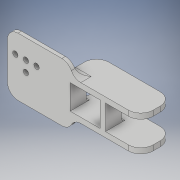
# Autodesk Inventor part: v5_tibia_B
Saved by Autodesk Inventor 2019 (Build 230136000, 136)
## iProperties
Created: 2019-01-20
Part Number: v5_tibia_B
Material: Generic
Document SubType Name: Modeling
Designer: Daniel
Density: 1 g/cm^3
Appearance: Default
Author: Daniel
Autodesk Inventor part; units mm, degrees
ref_plane "YZ Plane" through (0, 0, 0) normal (1, 0, 0) x (0, 1, 0)
ref_plane "XZ Plane" through (0, 0, 0) normal (0, 1, 0) x (-1, 0, 0)
ref_plane "XY Plane" through (0, 0, 0) normal (0, 0, 1) x (1, 0, 0)
sketch "Sketch1" plane through (0, 0, 0) normal (0, 1, 0) x (-1, 0, 0)
  line L0 (39, 2) -> (-3, 2)
  line L1 (-3, 2) -> (-3, 0)
  line L2 (-3, 0) -> (39, 0)
  line L3 (39, 0) -> (39, 2)
  line L4 (47.4, 0) -> (-11.4, 0) projected
  line L5 (0, -19.6) -> (0, 5.6) projected
  line L6 (0, -16) -> (-3, -16)
  line L7 (-3, -16) -> (-3, 0)
  line L8 (-3, 0) -> (0, 0)
  line L9 (0, 0) -> (0, -16)
  point P0 (0, 0)
  dimension "d0" = 2
  dimension "d1" = 3
  dimension "d2" = 42
  dimension "d3" = 18
  constraints: 16 end point, 4 collinear, 4 parallel, 2 horizontal, 2 perpendicular
  measures "d0" distance between parallel lines of L0 L2
  measures "d1" distance between parallel lines of L7 L9
  measures "d2" distance between parallel lines of L1 L3
  measures "d3" distance between parallel lines of L0 L6
extrude "Extrusion1" add sketch "Sketch1" along normal blind 33
sketch "Sketch2" plane through (-39, 0, 2) normal (0, 0, 1) x (1, 0, 0)
  line L0 (0, 0) -> (42, 0) projected
  line L1 (42, 0) -> (42, 33) projected
  line L2 (0, 33) -> (42, 33) projected
  line L3 (0, 0) -> (0, 33) projected
  point P0 (39, 0)
  point P1 (17, 11)
  point P2 (17, 17)
  point P3 (11, 11)
  point P4 (23, 11)
  dimension "d7" = 6
  dimension "d8" = 6
  dimension "d9" = 6
  dimension "d11" = 11
  dimension "d12" = 6
  dimension "d14" = 6
  dimension "d15" = 6
  dimension "d69" = 11
  measures "d7" distance of point (17, 11) point (17, 17)
  measures "d8" distance of point (17, 11) point (11, 11)
  measures "d9" distance of point (17, 11) point (23, 11)
  measures "d11" distance from line of L3 point (11, 11)
  measures "d12" horizontal distance of point (17, 17) point (11, 11)
  measures "d14" horizontal distance of point (17, 17) point (23, 11)
  measures "d15" horizontal distance of point (11, 11) point (17, 17)
  measures "d69" distance from line of L0 point (11, 11)
hole "Hole1" at (-22, 11, 2) at (-22, 17, 2) at (-28, 11, 2) at (-16, 11, 2) direction (0, 0, -1) diameter 3 end through all
sketch "Sketch9" plane through (3, 0, 2) normal (1, 0, 0) x (0, 0, -1)
  line L0 (18, 0) -> (0, 0) projected
  line L1 (18, 0) -> (18, 33) projected
  line L2 (0, 33) -> (18, 33) projected
  line L3 (0, 0) -> (0, 33) projected
  line L4 (2, 0) -> (2, 33) projected
  line L5 (0, 0) -> (0, 33) projected
  line L6 (0, 16.5) -> (18, 16.5) construction
  line L7 (0, 6.5) -> (18, 6.5)
  line L8 (18, 6.5) -> (18, 9.5)
  line L9 (18, 9.5) -> (0, 9.5)
  line L10 (0, 9.5) -> (0, 6.5)
  line L11 (0, 23.5) -> (18, 23.5)
  line L12 (18, 23.5) -> (18, 26.5)
  line L13 (18, 26.5) -> (0, 26.5)
  line L14 (0, 26.5) -> (0, 23.5)
  line L15 (0, 0) -> (0, 33) projected
  line L16 (18, 0) -> (18, 33) projected
  dimension "d81" = 16.5
  dimension "d82" = 3
  dimension "d83" = 3
  dimension "d84" = 7
  dimension "d85" = 7
  constraints: 18 end point, 4 parallel, 3 collinear, 3 perpendicular, 2 horizontal, 2 midpoint, 1 point on line
  measures "d81" distance between parallel lines of L2 L6
  measures "d82" distance between parallel lines of L13 L11
  measures "d83" distance between parallel lines of L7 L9
  measures "d84" distance between parallel lines of L6 L9
  measures "d85" distance between parallel lines of L11 L6
extrude "Extrusion6" add sketch "Sketch9" along normal blind 40 contours L7 L4 L9 L1 | L7 L3 L9 L4 | L11 L4 L13 L1 | L11 L3 L13 L4
sketch "Sketch10" plane through (3, 33, 2) normal (1, 0, 0) x (0, 0, -1)
  line L0 (18, -26.5) -> (0, -26.5) projected
  line L1 (0, -33) -> (0, -26.5) projected
  line L2 (18, -33) -> (0, -33) projected
  line L3 (18, -33) -> (18, -26.5) projected
  line L4 (0, -6.5) -> (18, -6.5) projected
  line L5 (18, -6.5) -> (18, 0) projected
  line L6 (0, 0) -> (18, 0) projected
  line L7 (0, -6.5) -> (0, 0) projected
  line L8 (0, -26.5) -> (18, -26.5) projected
  line L9 (18, -33) -> (2, -33)
  line L10 (2, -33) -> (2, -26.5)
  line L11 (2, -26.5) -> (18, -26.5)
  line L12 (18, -26.5) -> (18, -33)
  line L13 (18, -6.5) -> (0, -6.5) projected
  line L14 (18, 0) -> (2, 0)
  line L15 (2, 0) -> (2, -6.5)
  line L16 (2, -6.5) -> (18, -6.5)
  line L17 (18, -6.5) -> (18, 0)
  line L18 (2, -33) -> (2, 0) projected
  constraints: 16 end point, 4 parallel, 3 point on line, 2 horizontal, 2 perpendicular, 1 collinear
extrude "Extrusion7" cut sketch "Sketch10" against normal up to next contours L3 L2 L10 L0 | L15 L6 L5 L4
sketch "Sketch11" plane through (3, 9.5, 2) normal (0, 1, 0) x (1, 0, 0)
  line L0 (-3, 18) -> (-3, 2) projected
  line L1 (40, 18) -> (-3, 18) projected
  line L2 (40, 0) -> (40, 18) projected
  line L3 (0, 0) -> (40, 0) projected
  line L4 (17, 0) -> (20, 0)
  line L5 (20, 0) -> (20, 18)
  line L6 (20, 18) -> (17, 18)
  line L7 (17, 18) -> (17, 0)
  line L8 (0, 2) -> (-3, 2) projected
  line L9 (0, 2) -> (0, 0) projected
  point P0 (-3, 2)
  dimension "d92" = 3
  dimension "d97" = 20
  constraints: 8 end point, 2 collinear, 2 parallel, 1 horizontal, 1 perpendicular
  measures "d92" distance between parallel lines of L7 L5
  measures "d97" distance between parallel lines of L2 L5
extrude "Extrusion8" add sketch "Sketch11" along normal up to next contours L1 L5 L3 L7
fillet "Fillet18" radius 7 5 edges at (43, 25, 2) (43, 8, 2) (43, 25, -16) (43, 8, -16) (0, 16.5, -16)
sketch "Sketch15" plane through (23, 9.5, 2) normal (1, 0, 0) x (0, 0, -1)
  line L0 (0, 14) -> (18, 14) projected
  line L1 (0, 0) -> (0, 14) projected
  line L2 (18, 0) -> (0, 0) projected
  line L3 (18, 0) -> (18, 14) projected
  line L4 (0, 0) -> (16.7446, 0) projected
  line L5 (18, 14) -> (9, 14)
  line L6 (9, 14) -> (9, 0)
  line L7 (9, 0) -> (18, 0)
  line L8 (18, 0) -> (18, 14)
  point P0 (2, -9.5)
  dimension "d105" = 9
  constraints: 8 end point, 2 collinear, 2 parallel, 1 horizontal, 1 perpendicular, 1 point on line
  measures "d105" distance between parallel lines of L1 L6
extrude "Extrusion10" cut sketch "Sketch15" against normal through all contours L0 L3 L2 L6
fillet "Fillet23" radius 2 4 edges at (21.5, 9.5, -7) (21.5, 23.5, -7) (1.5, 23.5, -7) (1.5, 9.5, -7)
fillet "Fillet24" radius 4 3 edges at (1.5, 26.5, 0) (1.5, 6.5, 0) (0, 16.5, 0)
sketch "Sketch16" plane through (0, 33, 0) normal (0, 1, 0) x (1, 0, 0)
  line L0 (3, 0) -> (-39, 0) projected
  line L1 (-39, 0) -> (-39, -2) projected
  line L2 (-39, -2) -> (3, -2) projected
  line L3 (3, -2) -> (3, 0) projected
  line L4 (-29.5, 0) -> (-29.5, -2) projected
  line L5 (-23.5, 0) -> (-23.5, -2) projected
  line L6 (-17.5, 0) -> (-17.5, -2) projected
  line L7 (-14.5, 0) -> (-14.5, -2) projected
  line L8 (-26.5, 0) -> (-26.5, -2) projected
  line L9 (-20.5, 0) -> (-20.5, -2) projected
  line L10 (-17.5, 0) -> (-17.5, -2) projected
  line L11 (-39, 0) -> (-39, -2) projected
  line L12 (-39, -2) -> (3, -2) projected
  line L13 (-39, 0) -> (-32.5, 0)
  line L14 (-32.5, 0) -> (-32.5, -2)
  line L15 (-32.5, -2) -> (-39, -2)
  line L16 (-39, -2) -> (-39, 0)
  point P0 (0, 0)
  dimension "d110" = 3
  constraints: 8 end point, 2 parallel, 1 horizontal, 1 perpendicular, 4 other
  measures "d110" distance between parallel lines of L4 L14
extrude "Extrusion11" cut sketch "Sketch16" against normal up to next contours L14 L2 L1 L0
fillet "Fillet25" radius 6 6 edges at (-32.5, 33, 1) (3, 33, 1) (3, 26.5, -1) (3, 0, 1) (3, 6.5, -1) (-32.5, 0, 1)
mirror "Mirror1" about plane through (0, 0, 0) normal (0, 1, 0) remove original yes
body "Solid1"
